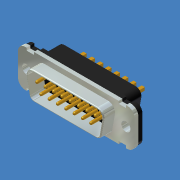
# Autodesk Inventor part: DBConnector
Saved by Autodesk Inventor 2019 (Build 230136000, 136)
## iProperties
Shininess: 64.0
Angle Display Precision: 2
Document Length Units: 11272
Document Angle Units: 11279
Document Time Units: 11290
Document Mass Units: 11286
Document Length Units Precision: 3
Document Angle Units Precision: 2
Compacted: True
Created: 2001-12-01
Part Number: DBConnector
Description: Dsub 15 Pin, 2 Row, Male
Document SubType Name: Modeling
Designer: Charles Bliss
Material: Generic
Density: 1 g/cm^3
Appearance: Zinc
Density: 0.0
Volumn: 0.0
Area: 0.0
PropertySet Name: Model Information
Control State: 0
Master: False
Checked Out: False
Author: Charles Bliss
Autodesk Inventor part; units mm, degrees
ref_plane "YZ Plane" through (0, 0, 0) normal (1, 0, 0) x (0, 1, 0)
ref_plane "XZ Plane" through (0, 0, 0) normal (0, 1, 0) x (-1, 0, 0)
ref_plane "XY Plane" through (0, 0, 0) normal (0, 0, 1) x (1, 0, 0)
sketch "Sketch1" plane through (0, 0, 0) normal (0, 0, 1) x (1, 0, 0)
  line L0 (-14.244, 6.2738) -> (14.244, 6.2738)
  line L1 (14.244, 6.2738) -> (14.244, 5.4179)
  line L2 (14.244, 5.4179) -> (16.6624, 5.4179)
  line L3 (16.6624, 5.4179) -> (16.6624, 6.2738)
  line L4 (16.6624, 6.2738) -> (17.1523, 6.2738)
  arc A0 (19.5707, 3.8554) -> (17.1523, 6.2738) centre (17.1523, 3.8554) ccw
  line L5 (-14.244, 6.2738) -> (-14.244, 5.4179)
  line L6 (-14.244, 5.4179) -> (-16.6624, 5.4179)
  line L7 (-16.6624, 5.4179) -> (-16.6624, 6.2738)
  line L8 (-16.6624, 6.2738) -> (-17.1523, 6.2738)
  arc A1 (-17.1523, 6.2738) -> (-19.5707, 3.8554) centre (-17.1523, 3.8554) ccw
  line L9 (-19.5707, 0) -> (19.5707, 0) construction
  line L10 (-14.244, -6.2738) -> (14.244, -6.2738)
  line L11 (-14.244, -6.2738) -> (-14.244, -5.4179)
  line L12 (-14.244, -5.4179) -> (-16.6624, -5.4179)
  line L13 (-16.6624, -5.4179) -> (-16.6624, -6.2738)
  line L14 (-16.6624, -6.2738) -> (-17.1523, -6.2738)
  arc A2 (-19.5707, -3.8554) -> (-17.1523, -6.2738) centre (-17.1523, -3.8554) ccw
  line L15 (14.244, -6.2738) -> (14.244, -5.4179)
  line L16 (14.244, -5.4179) -> (16.6624, -5.4179)
  line L17 (16.6624, -5.4179) -> (16.6624, -6.2738)
  line L18 (16.6624, -6.2738) -> (17.1523, -6.2738)
  arc A3 (17.1523, -6.2738) -> (19.5707, -3.8554) centre (17.1523, -3.8554) ccw
  line L19 (-19.5707, 3.8554) -> (-19.5707, -3.8554)
  line L20 (19.5707, 3.8554) -> (19.5707, -3.8554)
  line L21 (-12.0832, -3.1583) -> (-12.97, 1.8711)
  arc A4 (-10.7144, 4.5593) -> (-12.97, 1.8711) centre (-10.7144, 2.2689) ccw
  line L22 (-10.7144, 4.5593) -> (10.7144, 4.5593)
  arc A5 (12.97, 1.8711) -> (10.7144, 4.5593) centre (10.7144, 2.2689) ccw
  line L23 (12.97, 1.8711) -> (12.0832, -3.1583)
  arc A6 (10.4135, -4.5593) -> (12.0832, -3.1583) centre (10.4135, -2.8639) ccw
  line L24 (10.4135, -4.5593) -> (-10.4135, -4.5593)
  arc A7 (-12.0832, -3.1583) -> (-10.4135, -4.5593) centre (-10.4135, -2.8639) ccw
  line L25 (0, 6.2738) -> (0, -6.2738) construction
  line L26 (0, 4.5593) -> (0, -4.5593) construction
  line L27 (-10.4135, -4.1783) -> (10.4135, -4.1783)
  arc A8 (10.4135, -4.1783) -> (11.708, -3.0921) centre (10.4135, -2.8639) ccw
  line L28 (11.708, -3.0921) -> (12.5948, 1.9373)
  arc A9 (12.5948, 1.9373) -> (10.7144, 4.1783) centre (10.7144, 2.2689) ccw
  line L29 (10.7144, 4.1783) -> (-10.7144, 4.1783)
  arc A10 (-10.7144, 4.1783) -> (-12.5948, 1.9373) centre (-10.7144, 2.2689) ccw
  line L30 (-12.5948, 1.9373) -> (-11.708, -3.0921)
  arc A11 (-11.708, -3.0921) -> (-10.4135, -4.1783) centre (-10.4135, -2.8639) ccw
  circle A12 centre (-16.6624, 0) radius 1.524
  circle A13 centre (16.6624, 0) radius 1.524
  line L31 (-16.6624, 0) -> (0, 0) construction
  line L32 (0, 0) -> (16.6624, 0) construction
  line L33 (12.6238, 6.2738) -> (12.6238, 2.2689) construction
  line L34 (-12.6238, 6.2738) -> (-12.6238, 2.2689) construction
  line L35 (-12.8909, 1.4224) -> (12.8909, 1.4224) construction
  line L36 (-12.3893, -1.4224) -> (12.3893, -1.4224) construction
  circle A14 centre (-9.779, 1.4224) radius 0.4953
  circle A15 centre (-8.382, -1.4224) radius 0.4953
  line L37 (-11.8877, -4.2672) -> (11.8877, -4.2672) construction
  circle A16 centre (-9.779, -4.2672) radius 0.4953
  point P0 (0, -1.4224)
  dimension "d0" = 10
  dimension "HoleCtr" = 33.3248
  dimension "OAL" = 39.1414
  dimension "ShellLen" = 25.2476
  dimension "ShellWid" = 8.3566
  dimension "HoleDia" = 3.048
  dimension "d6" = 0.381
  dimension "d7" = 2.4184
  dimension "d8" = 0.8559
  dimension "d9" = 2.4184
  dimension "OAW" = 12.5476
  dimension "d11" = 1.3144
  dimension "PinVertDist" = 2.8448
  dimension "PinDia" = 0.9906
  dimension "Pin1Offset" = 9.779
  dimension "d19" = 1.397
  dimension "d34" = 1.9094
  dimension "CLoffset" = 2.7559
  dimension "d52" = 2.8448
  constraints: 76 end point, 26 point on circle, 17 centre point, 16 tangent, 14 point on line, 14 symmetric about line, 10 parallel, 8 midpoint, 6 equal length, 6 equal radius, 5 collinear, 4 perpendicular, 3 horizontal, 3 vertical alignment, 2 coincident, 2 vertical, 18 other
  measures "d0" angle of L21 L19
  measures "HoleCtr" diameter of A12.centre L25
  measures "OAL" distance between parallel lines of L20 L19
  measures "ShellLen" distance between parallel lines of L33 L34
  measures "ShellWid" distance between parallel lines of L27 L29
  measures "HoleDia" diameter of A13
  measures "d6" distance between parallel lines of L30 L21
  measures "d7" distance of L6.start L6.end
  measures "d8" distance of L0.start L6.start
  measures "d9" radius of A1
  measures "OAW" distance between parallel lines of L10 L0
  measures "d11" radius of A8
  measures "PinVertDist" distance between parallel lines of L36 L35
  measures "PinDia" diameter of A15
  measures "Pin1Offset" distance from line of A14.centre L26
  measures "d19" horizontal distance of A15.centre A14.centre
  measures "d34" radius of A10
  measures "CLoffset" distance between parallel lines of L27 L36
  measures "d52" distance between parallel lines of L37 L36
extrude "Extrusion1" add sketch "Sketch1" along normal blind 1.27 contours L0 L1 L2 L3 L4 A0 L20 A3 L18 L17 L16 L15 L10 L11 L12 L13 L14 A2 L19 A1 L8 L7 L6 L5 | L21 A4 L22 A5 L23 A6 L24 A16 L27 A8 L28 A9 L29 A10 L30 A11 A7 | A16 L27 L24 | L24 A16
extrude "Extrusion2" add sketch "Sketch1" along normal blind 5.08 contours L21 A4 L22 A5 L23 A6 L24 A16 L27 A8 L28 A9 L29 A10 L30 A11 A7 | A16 L27 L24
fillet "Fillet4" radius 0.381 8 edges at (-11.5033, -4.1626, 5.08) (-12.5266, -0.6436, 5.08) (-12.4689, 3.7411, 5.08) (0, 4.5593, 5.08) (12.4689, 3.7411, 5.08) (12.5266, -0.6436, 5.08) (11.5033, -4.1626, 5.08) (0, -4.5593, 5.08)
extrude "Pin1" add sketch "Sketch1" along normal blind 5.08 contours A14
extrude "Pin2" add sketch "Sketch1" along normal blind 5.08 contours A15
extrude "Pin50" [suppressed]
fillet "Fillet1" radius 0.4953 1 edges at (-10.2743, 1.4224, 5.08)
fillet "Fillet2" radius 0.4953 1 edges at (-8.8773, -1.4224, 5.08)
fillet "Fillet50" [suppressed]
sketch "Sketch2" plane through (0, 0, 0) normal (0, 0, -1) x (-1, 0, 0)
  circle A0 centre (-16.6624, 0) radius 1.524 projected
  circle A1 centre (16.6624, 0) radius 1.524 projected
  line L0 (14.244, 6.2738) -> (-14.244, 6.2738) projected
  line L1 (-14.244, 6.2738) -> (-14.244, 5.4179) projected
  line L2 (-14.244, 5.4179) -> (-16.6624, 5.4179) projected
  line L3 (-16.6624, 5.4179) -> (-16.6624, 6.2738) projected
  line L4 (-16.6624, 6.2738) -> (-17.1523, 6.2738) projected
  arc A2 (-17.1523, 6.2738) -> (-19.5707, 3.8554) centre (-17.1523, 3.8554) ccw projected
  line L5 (-19.5707, 3.8554) -> (-19.5707, -3.8554) projected
  arc A3 (-19.5707, -3.8554) -> (-17.1523, -6.2738) centre (-17.1523, -3.8554) ccw projected
  line L6 (-17.1523, -6.2738) -> (-16.6624, -6.2738) projected
  line L7 (-16.6624, -6.2738) -> (-16.6624, -5.4179) projected
  line L8 (-16.6624, -5.4179) -> (-14.244, -5.4179) projected
  line L9 (-14.244, -5.4179) -> (-14.244, -6.2738) projected
  line L10 (-14.244, -6.2738) -> (14.244, -6.2738) projected
  line L11 (14.244, -6.2738) -> (14.244, -5.4179) projected
  line L12 (14.244, -5.4179) -> (16.6624, -5.4179) projected
  line L13 (16.6624, -5.4179) -> (16.6624, -6.2738) projected
  line L14 (16.6624, -6.2738) -> (17.1523, -6.2738) projected
  arc A4 (17.1523, -6.2738) -> (19.5707, -3.8554) centre (17.1523, -3.8554) ccw projected
  line L15 (19.5707, -3.8554) -> (19.5707, 3.8554) projected
  arc A5 (19.5707, 3.8554) -> (17.1523, 6.2738) centre (17.1523, 3.8554) ccw projected
  line L16 (17.1523, 6.2738) -> (16.6624, 6.2738) projected
  line L17 (16.6624, 6.2738) -> (16.6624, 5.4179) projected
  line L18 (16.6624, 5.4179) -> (14.244, 5.4179) projected
  line L19 (14.244, 5.4179) -> (14.244, 6.2738) projected
  line L20 (-13.99, 6.0198) -> (13.99, 6.0198)
  line L21 (13.99, 6.0198) -> (13.99, 5.1639)
  line L22 (13.99, 5.1639) -> (16.9164, 5.1639)
  line L23 (16.9164, 5.1639) -> (16.9164, 6.0198)
  line L24 (16.9164, 6.0198) -> (17.1523, 6.0198)
  arc A6 (19.3167, 3.8554) -> (17.1523, 6.0198) centre (17.1523, 3.8554) ccw
  line L25 (19.3167, 3.8554) -> (19.3167, -3.8554)
  arc A7 (17.1523, -6.0198) -> (19.3167, -3.8554) centre (17.1523, -3.8554) ccw
  line L26 (17.1523, -6.0198) -> (16.9164, -6.0198)
  line L27 (16.9164, -6.0198) -> (16.9164, -5.1639)
  line L28 (16.9164, -5.1639) -> (13.99, -5.1639)
  line L29 (13.99, -5.1639) -> (13.99, -6.0198)
  line L30 (13.99, -6.0198) -> (-13.99, -6.0198)
  line L31 (-13.99, -6.0198) -> (-13.99, -5.1639)
  line L32 (-13.99, -5.1639) -> (-16.9164, -5.1639)
  line L33 (-16.9164, -5.1639) -> (-16.9164, -6.0198)
  line L34 (-16.9164, -6.0198) -> (-17.1523, -6.0198)
  arc A8 (-19.3167, -3.8554) -> (-17.1523, -6.0198) centre (-17.1523, -3.8554) ccw
  line L35 (-19.3167, -3.8554) -> (-19.3167, 3.8554)
  arc A9 (-17.1523, 6.0198) -> (-19.3167, 3.8554) centre (-17.1523, 3.8554) ccw
  line L36 (-17.1523, 6.0198) -> (-16.9164, 6.0198)
  line L37 (-16.9164, 6.0198) -> (-16.9164, 5.1639)
  line L38 (-16.9164, 5.1639) -> (-13.99, 5.1639)
  line L39 (-13.99, 5.1639) -> (-13.99, 6.0198)
  dimension "d35" = 0.254
  constraints: 40 end point, 8 point on circle, 4 centre point, 23 other
  measures "d35" distance between parallel lines of L5 L35
extrude "Extrusion5" add sketch "Sketch2" along normal blind 1.6002 contours L20 L21 L22 L23 L24 A6 L25 A7 L26 L27 L28 L29 L30 L31 L32 L33 L34 A8 L35 A9 L36 L37 L38 L39
sketch "Sketch3" plane through (0, 0, -1.6002) normal (0, 0, -1) x (-1, 0, 0)
  line L0 (-12.0134, 5.4483) -> (12.0134, 5.4483)
  arc A0 (13.8938, 3.2073) -> (12.0134, 5.4483) centre (12.0134, 3.5389) ccw
  line L1 (13.8938, 3.2073) -> (12.6458, -3.8704)
  arc A1 (10.7654, -5.4483) -> (12.6458, -3.8704) centre (10.7654, -3.5389) ccw
  line L2 (10.7654, -5.4483) -> (-10.7654, -5.4483)
  arc A2 (-12.6458, -3.8704) -> (-10.7654, -5.4483) centre (-10.7654, -3.5389) ccw
  line L3 (-12.6458, -3.8704) -> (-13.8938, 3.2073)
  arc A3 (-12.0134, 5.4483) -> (-13.8938, 3.2073) centre (-12.0134, 3.5389) ccw
  line L4 (0, 0) -> (0, 5.4483) construction
  line L5 (0, 0) -> (0, -5.4483) construction
  line L6 (-13.99, 6.0198) -> (13.99, 6.0198) projected
  line L7 (-12.97, 1.8711) -> (-12.0832, -3.1583) projected
  dimension "d86" = 1.9094
  dimension "d87" = 10.8966
  dimension "d88" = 27.7876
  constraints: 12 end point, 8 point on circle, 8 tangent, 4 centre point, 2 equal length, 2 horizontal alignment, 2 midpoint, 2 vertical, 1 equal radius, 1 parallel, 1 perpendicular
  measures "d86" radius of A2
  measures "d87" distance of L5.end L4.end
  measures "d88" distance of L1.start L3.end
extrude "Extrusion6" add sketch "Sketch3" along normal blind 5.08
sketch "Sketch4" plane through (0, 0, -6.6802) normal (0, 0, -1) x (-1, 0, 0)
  line L0 (7.874, -0.9144) -> (8.89, -0.9144)
  line L1 (8.89, -0.9144) -> (8.89, -1.9304)
  line L2 (8.89, -1.9304) -> (7.874, -1.9304)
  line L3 (7.874, -1.9304) -> (7.874, -0.9144)
  line L4 (9.271, 1.9304) -> (10.287, 1.9304)
  line L5 (10.287, 1.9304) -> (10.287, 0.9144)
  line L6 (10.287, 0.9144) -> (9.271, 0.9144)
  line L7 (9.271, 0.9144) -> (9.271, 1.9304)
  line L8 (10.287, -4.7752) -> (9.271, -4.7752)
  line L9 (9.271, -4.7752) -> (9.271, -3.7592)
  line L10 (9.271, -3.7592) -> (10.287, -3.7592)
  line L11 (10.287, -3.7592) -> (10.287, -4.7752)
  point P0 (9.779, 1.4224)
  point P1 (8.382, -1.4224)
  point P2 (8.382, -1.4224)
  point P3 (9.779, 1.4224)
  point P4 (9.779, -4.2672)
  point P5 (9.779, -4.2672)
  dimension "d46" = 1.016
  constraints: 24 end point, 3 coincident, 3 horizontal, 2 parallel, 21 other
  measures "d46" distance of L4.end L5.end
extrude "ExtrudeSgr50" [suppressed]
chamfer "Chamfer50" [suppressed]
pattern_linear "Pattern1" count 8 spacing 2.794 along (1, 0, 0) of "Pin1", "Fillet1"
pattern_linear "Pattern2" count 7 spacing 2.794 along (1, 0, 0) of "Pin2", "Fillet2"
pattern_linear "Pattern50" [suppressed]
extrude "Female" [suppressed]
extrude "Socket1" [suppressed]
extrude "Socket2" [suppressed]
extrude "Socket50" [suppressed]
pattern_linear "Pattern5" [suppressed]
pattern_linear "Pattern6" [suppressed]
pattern_linear "Pattern7" [suppressed]
equation "\"d19\" = 0.5 * PinSpace"
equation "\"d52\" = PinVertDist"
equation "\"d63\" = d6"
equation "\"d26\" = d24"
equation "\"d53\" = d24"
equation "\"d44\" = 0.5 * PinDia"
equation "\"d45\" = 0.5 * PinDia"
equation "\"d55\" = 0.5 * PinDia"
equation "\"d56\" = d24"
equation "\"d58\" = 0.2 * d46"
equation "\"d59\" = 0.2 * d46"
equation "\"d30\" = PinSpace"
equation "\"d33\" = PinSpace"
equation "\"d62\" = PinSpace"
equation "\"d77\" = PinSpace"
equation "\"d80\" = PinSpace"
equation "\"d83\" = PinSpace"
equation "\"PinSpace\" = 2.794"
equation "\"RowOffset\" = 1.397"
equation "\"d24\" = 5.08"
body "Solid1"
